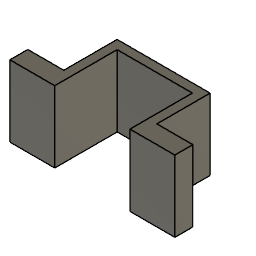
mocowanie_silnik (Autodesk Fusion 360 design; units mm, degrees)
part number: 2025-11-29-23-35-01-223
Autodesk Fusion 360 part; units mm, degrees
sketch "Szkic1" plane through (0, 0, 0) normal (0, 0, 1) x (1, 0, 0)
  line L0 (0, 0) -> (0, 2.9)
  line L1 (0, 2.9) -> (5.8, 2.9)
  line L2 (5.8, 2.9) -> (5.8, 11.5)
  line L3 (5.8, 11.5) -> (20.8, 11.5)
  line L4 (20.8, 11.5) -> (20.8, 2.9)
  line L5 (20.8, 2.9) -> (26.6, 2.9)
  line L6 (26.6, 2.9) -> (26.6, 0)
  line L7 (26.6, 0) -> (19.36, 0)
  line L8 (19.36, 0) -> (19.36, 10.06)
  line L9 (19.36, 10.06) -> (7.24, 10.06)
  line L10 (7.24, 10.06) -> (7.24, 0)
  line L11 (7.24, 0) -> (0, 0)
  dimension "d1" = 2.9
  dimension "d2" = 5.8
  dimension "d3" = 8.6
  dimension "d4" = 15
  dimension "d5" = 8.6
  dimension "d6" = 5.8
  dimension "d7" = 7.24
  dimension "d8" = 10.06
  dimension "d9" = 12.12
  dimension "d10" = 10.06
  constraint vertical L0
  constraint coincident L0.start L11.end
  constraint perpendicular L0 L1
  constraint perpendicular L1 L2
  constraint perpendicular L2 L3
  constraint perpendicular L3 L4
  constraint perpendicular L4 L5
  constraint perpendicular L5 L6
  constraint perpendicular L6 L7
  constraint perpendicular L7 L8
  constraint perpendicular L8 L9
  constraint perpendicular L9 L10
  constraint perpendicular L0 L11
  measures "d1" distance of L0.start L0.end
  measures "d2" distance of L0.end L1.end
  measures "d3" distance of L1.end L2.end
  measures "d4" distance of L2.end L3.end
  measures "d5" distance of L3.end L4.end
  measures "d6" distance of L4.end L5.end
  measures "d7" distance of L6.end L7.end
  measures "d8" distance of L7.end L8.end
  measures "d9" distance of L8.end L9.end
  measures "d10" distance of L9.end L10.end
extrude "Wyciągnięcie proste1" add sketch "Szkic1" along normal blind 11.5
